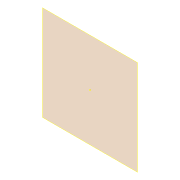
# Autodesk Inventor part: 10_Baseplate_axiotech
Saved by Autodesk Inventor 2019 (Build 230136000, 136)
## iProperties
Created: 2019-05-21
Part Number: 10_Baseplate_axiotech
Material: Generic
Document SubType Name: Modeling
Designer: diederichbenedict
Density: 1 g/cm^3
Appearance: Default
Author: diederichbenedict
Autodesk Inventor part; units mm, degrees
ref_plane "YZ Plane" through (0, 0, 0) normal (1, 0, 0) x (0, 1, 0)
ref_plane "XZ Plane" through (0, 0, 0) normal (0, 1, 0) x (-1, 0, 0)
ref_plane "XY Plane" through (0, 0, 0) normal (0, 0, 1) x (1, 0, 0)
ref_plane "Work Plane1" through (0, 0, 0) normal (0, 0, 1) x (1, 0, 0)
sketch "Sketch1" plane through (0, 0, 0) normal (0, 0, 1) x (1, 0, 0)
  circle A0 centre (0, 25) radius 1.95 construction
  circle A1 centre (-25, 0) radius 1.95 construction
  circle A2 centre (-25, -25) radius 1.95 construction
  circle A3 centre (25, 25) radius 1.95 construction
  circle A4 centre (25, -25) radius 1.95 construction
  circle A5 centre (-25, 25) radius 1.95 construction
  circle A6 centre (25, 0) radius 1.95 construction
  circle A7 centre (0, -25) radius 1.95 construction
  line L0 (-28, 30) -> (-30, 28) construction
  line L1 (-30, 28) -> (-30, -28) construction
  line L2 (-30, -28) -> (-28, -30) construction
  line L3 (-28, -30) -> (28, -30) construction
  line L4 (28, -30) -> (30, -28) construction
  line L5 (30, -28) -> (30, 28) construction
  line L6 (30, 28) -> (28, 30) construction
  line L7 (28, 30) -> (-28, 30) construction
  circle A8 centre (-145, 0) radius 1.95 construction
  circle A9 centre (-120, -25) radius 1.95 construction
  circle A10 centre (-95, -25) radius 1.95 construction
  circle A11 centre (-145, 25) radius 1.95 construction
  circle A12 centre (-95, 25) radius 1.95 construction
  circle A13 centre (-145, -25) radius 1.95 construction
  circle A14 centre (-120, 25) radius 1.95 construction
  circle A15 centre (-95, 0) radius 1.95 construction
  line L8 (-150, -28) -> (-148, -30) construction
  line L9 (-148, -30) -> (-92, -30) construction
  line L10 (-92, -30) -> (-90, -28) construction
  line L11 (-90, -28) -> (-90, 28) construction
  line L12 (-90, 28) -> (-92, 30) construction
  line L13 (-92, 30) -> (-148, 30) construction
  line L14 (-148, 30) -> (-150, 28) construction
  line L15 (-150, 28) -> (-150, -28) construction
  line L16 (-150, 29.9315) -> (29.9315, 29.9315)
  line L17 (29.9315, 29.9315) -> (29.9315, -30)
  line L18 (29.9315, -30) -> (-150, -30)
  line L19 (-150, -30) -> (-150, 29.9315)
  circle A16 centre (-145, 25) radius 1.95 construction
  circle A17 centre (-120, 25) radius 1.95 construction
  point P0 (0, 0)
  constraints: 8 end point, 2 parallel, 1 horizontal, 1 perpendicular, 1 point on line
extrude "Extrusion1" add sketch "Sketch1" along normal blind 17
sketch "Sketch2" plane through (0, 0, 17) normal (0, 0, 1) x (1, 0, 0)
  line L0 (-81.5, -37.6742) -> (-81.5, -40.2723) construction
  line L1 (-81.5, -40.2723) -> (-79.9, -40.2723) construction
  line L2 (-79.9, -40.2723) -> (-79.9, -52.9723) construction
  line L3 (-79.9, -52.9723) -> (-83, -52.9723) construction
  line L4 (-83, -53.9723) -> (-83, -52.9723) construction
  line L5 (-83, -53.9723) -> (-76.1, -53.9723) construction
  line L6 (-76.1, -53.9723) -> (-76.1, -67.5723) construction
  line L7 (-76.1, -67.5723) -> (-83, -67.5723) construction
  line L8 (-83, -69.7723) -> (-83, -67.5723) construction
  line L9 (-83, -69.7723) -> (-74.45, -69.7723) construction
  line L10 (-74.45, -69.7723) -> (-74.45, -66.4223) construction
  line L11 (-74.45, -66.4223) -> (-65.85, -66.4223) construction
  line L12 (-65.85, -66.4223) -> (-65.85, -71.4223) construction
  line L13 (-65.85, -71.4223) -> (-70, -71.4223) construction
  line L14 (-70, -74.1723) -> (-70, -71.4223) construction
  arc A0 (-70, -74.1723) -> (-51.8, -75.6302) centre (-59.1233, -52.722) ccw construction
  line L15 (-51.8, -75.6302) -> (-51.8, -70.6223) construction
  line L16 (-51.8, -70.6223) -> (-56.55, -70.6223) construction
  line L17 (-56.55, -70.6223) -> (-56.55, -73.8223) construction
  arc A1 (-57.55, -74.8223) -> (-56.55, -73.8223) centre (-57.55, -73.8223) ccw construction
  line L18 (-57.55, -74.8223) -> (-64.05, -74.8223) construction
  arc A2 (-65.05, -73.8223) -> (-64.05, -74.8223) centre (-64.05, -73.8223) ccw construction
  line L19 (-65.05, -73.8223) -> (-66.55, -73.8223) construction
  line L20 (-66.55, -73.8223) -> (-66.55, -72.3223) construction
  line L21 (-66.55, -72.3223) -> (-65.05, -72.3223) construction
  line L22 (-65.05, -72.3223) -> (-65.05, -65.8223) construction
  line L23 (-65.05, -65.8223) -> (-66.05, -64.8223) construction
  line L24 (-66.05, -64.8223) -> (-74.5, -64.8223) construction
  line L25 (-74.5, -64.8223) -> (-74.5, -49.7723) construction
  arc A3 (-74.5, -49.7723) -> (-76.95, -47.3223) centre (-76.95, -49.7723) ccw construction
  line L26 (-76.95, -47.3223) -> (-78.2, -47.3223) construction
  arc A4 (-78.7, -46.8223) -> (-78.2, -47.3223) centre (-78.2, -46.8223) ccw construction
  line L27 (-78.7, -46.8223) -> (-78.7, -40.8223) construction
  arc A5 (-77.7, -39.8223) -> (-78.7, -40.8223) centre (-77.7, -40.8223) ccw construction
  line L28 (-77.7, -39.8223) -> (-76.1, -39.8223) construction
  line L29 (-76.1, -39.8223) -> (-76.1, -45.8223) construction
  arc A6 (-76.1, -45.8223) -> (-75.1, -46.8223) centre (-75.1, -45.8223) ccw construction
  line L30 (-75.1, -46.8223) -> (-74, -46.8223) construction
  arc A7 (-72, -48.8223) -> (-74, -46.8223) centre (-74, -48.8223) ccw construction
  line L31 (-72, -48.8223) -> (-72, -64.4223) construction
  line L32 (-72, -64.4223) -> (-63.75, -64.4223) construction
  line L33 (-63.75, -64.4223) -> (-62.3, -65.8723) construction
  line L34 (-62.3, -65.8723) -> (-62.3, -74.4223) construction
  line L35 (-62.3, -74.4223) -> (-60.3, -74.4223) construction
  line L36 (-60.3, -74.4223) -> (-60.3, -70.4223) construction
  line L37 (-60.3, -70.4223) -> (-48.75, -70.4223) construction
  line L38 (-48.75, -70.4223) -> (-48.75, -66.9223) construction
  line L39 (-48.75, -66.9223) -> (-47.75, -65.9223) construction
  line L40 (-42.8, -65.9223) -> (-47.75, -65.9223) construction
  line L41 (-42.8, -65.9223) -> (-42.8, -50.4723) construction
  line L42 (-42.8, -50.4723) -> (-33, -50.4723) construction
  line L43 (-33, -41.4723) -> (-33, -50.4723) construction
  line L44 (-35.8868, -36.4723) -> (-33, -41.4723) construction
  line L45 (-38, -36.4723) -> (-35.8868, -36.4723) construction
  line L46 (-38, -34.4723) -> (-38, -36.4723) construction
  line L47 (-38, -34.4723) -> (-54, -34.4723) construction
  line L48 (-54, -34.4723) -> (-54, -24.1723) construction
  line L49 (-54, -24.1723) -> (-57.2, -24.1723) construction
  line L50 (-57.2, -24.1723) -> (-57.2, -36.3723) construction
  line L51 (-57.2, -36.3723) -> (-57.7, -36.3723) construction
  line L52 (-57.7, -36.3723) -> (-58.7, -33.3723) construction
  line L53 (-58.7, -33.3723) -> (-58.7, -27.6723) construction
  line L54 (-58.7, -27.6723) -> (-61.7, -27.6723) construction
  line L55 (-61.7, -27.6723) -> (-61.7, -32.6723) construction
  line L56 (-61.7, -32.6723) -> (-62.7, -32.6723) construction
  arc A8 (-67.8, -36.4723) -> (-62.7, -32.6723) centre (-69.636, -28.6858) ccw construction
  line L57 (-80.8061, -36.4723) -> (-67.8, -36.4723) construction
  line L58 (-81.5, -37.6742) -> (-80.8061, -36.4723) construction
  line L59 (-60.7, -33.6723) -> (-60.7, -28.6723) construction
  line L60 (-60.7, -28.6723) -> (-59.7, -28.6723) construction
  line L61 (-59.7, -28.6723) -> (-59.7, -33.5346) construction
  line L62 (-59.7, -33.5346) -> (-58.7541, -36.3723) construction
  line L63 (-58.7541, -36.3723) -> (-64.9543, -36.3723) construction
  arc A9 (-64.9543, -36.3723) -> (-62.1437, -33.6723) centre (-69.636, -28.6858) ccw construction
  line L64 (-62.1437, -33.6723) -> (-60.7, -33.6723) construction
  circle A10 centre (-76.95, -49.7723) radius 1.45 construction
  arc A11 (-55, -60.3973) -> (-54, -61.3973) centre (-54, -60.3973) ccw construction
  line L65 (-55, -60.3973) -> (-55, -58.9473) construction
  line L66 (-55, -58.9473) -> (-66, -58.9473) construction
  line L67 (-66, -58.9473) -> (-66, -41.6473) construction
  arc A12 (-65, -40.6473) -> (-66, -41.6473) centre (-65, -41.6473) ccw construction
  line L68 (-65, -40.6473) -> (-62.5, -40.6473) construction
  arc A13 (-61.5, -41.6473) -> (-62.5, -40.6473) centre (-62.5, -41.6473) ccw construction
  line L69 (-61.5, -41.6473) -> (-61.5, -43.1473) construction
  line L70 (-61.5, -43.1473) -> (-50.8, -43.1473) construction
  line L71 (-50.8, -43.1473) -> (-50.8, -60.3973) construction
  arc A14 (-51.8, -61.3973) -> (-50.8, -60.3973) centre (-51.8, -60.3973) ccw construction
  line L72 (-51.8, -61.3973) -> (-54, -61.3973) construction
  line L73 (-37, -61.4723) -> (-37, -71) construction
  arc A15 (-51.8, -75.6302) -> (-44, -71.4223) centre (-59.1233, -52.722) ccw construction
  line L74 (-44, -65.9223) -> (-44, -71.4223) construction
  line L75 (-47.75, -65.9223) -> (-44, -65.9223) construction
  line L76 (-48.75, -66.9223) -> (-47.75, -65.9223) construction
  line L77 (-48.75, -70.4223) -> (-48.75, -66.9223) construction
  line L78 (-51.8, -70.4223) -> (-48.75, -70.4223) construction
  line L79 (-51.8, -75.6302) -> (-51.8, -70.4223) construction
  circle A16 centre (-46.1, -70.3914) radius 0.9 construction
  circle A17 centre (-73.1, -69.5223) radius 0.9 construction
  circle A18 centre (-67.85, -68.9223) radius 0.75 construction
  line L80 (-76.1, -69.7723) -> (-74.45, -69.7723) construction
  line L81 (-74.45, -71.4223) -> (-76.1, -69.7723) construction
  line L82 (-70, -71.4223) -> (-74.45, -71.4223) construction
  line L83 (-65.85, -71.4223) -> (-70, -71.4223) construction
  line L84 (-65.85, -66.4223) -> (-65.85, -71.4223) construction
  line L85 (-74.45, -66.4223) -> (-65.85, -66.4223) construction
  line L86 (-74.45, -69.7723) -> (-74.45, -66.4223) construction
  line L87 (-44, -74.4223) -> (-74.45, -74.4223) construction
  line L88 (-74.45, -74.4223) -> (-74.45, -30) construction
  line L89 (-74.45, -30) -> (-44, -30) construction
  line L90 (-44, -30) -> (-44, -74.4223) construction
  line L91 (-44, -74.4223) -> (-74.45, -74.4223)
  line L92 (-74.45, -74.4223) -> (-74.45, -30)
  line L93 (-74.45, -30) -> (-44, -30)
  line L94 (-44, -30) -> (-44, -74.4223)
  line L95 (-150, -30) -> (29.9315, -30) projected
  point P0 (0, 0)
  dimension "d7" = 0
  constraints: 16 end point, 4 parallel, 2 horizontal, 2 perpendicular
  measures "d7" distance between parallel lines of L89 L95
ref_plane "Work Plane2" through (-83, -76.7723, 14.1376) normal (0, 0, 1) x (1, 0, 0)
extrude "Extrusion2" add sketch "Sketch2" against normal up to surface (2.8624 mm away)
sketch "Sketch3" plane through (0, 0, 0) normal (0, 0, -1) x (-1, 0, 0)
  line L0 (44, -30) -> (44, -74.4223) projected
  line L1 (44, -74.4223) -> (74.45, -74.4223) projected
  line L2 (74.45, -74.4223) -> (74.45, -30) projected
  line L3 (44, -30) -> (74.45, -30) projected
  line L4 (44, -30) -> (74.45, -30) projected
  arc A0 (74.45, -30) -> (44, -30) centre (59.225, -30.3309) ccw
  point P0 (0, 0)
  constraints: 2 point on circle, 1 centre point
extrude "Extrusion3" cut sketch "Sketch3" against normal up to surface (14.1376 mm away)
body "Solid1"
